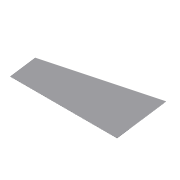
# Autodesk Inventor part: panelBflat_SA
Saved by Autodesk Inventor 2016 (Build 200138000, 138)
## iProperties
Created: 2015-02-12
Part Number: panelBflat_SA
Material: Generic
Document SubType Name: Modeling
Designer: Dave
Density: 1 g/cm^3
Appearance: Default
Author: Dave
Autodesk Inventor part; units mm, degrees
ref_plane "YZ Plane" through (0, 0, 0) normal (1, 0, 0) x (0, 1, 0)
ref_plane "XZ Plane" through (0, 0, 0) normal (0, 1, 0) x (-1, 0, 0)
ref_plane "XY Plane" through (0, 0, 0) normal (0, 0, 1) x (1, 0, 0)
sketch "Sketch1" plane through (0, 0, 0) normal (0, 1, 0) x (-1, 0, 0)
  line L0 (0, 0) -> (-4300, 0) construction
  line L1 (0, 0) -> (-4153.4811, -1112.9219) construction
  line L2 (0, 0) -> (4300, 0) construction
  line L3 (-4300, 0) -> (-4200, 0) construction
  line L4 (-2006.9086, 50) -> (-4293.6038, 50)
  line L5 (-4153.4811, -1112.9219) -> (-3780.7254, -1112.9219) construction
  line L6 (-1925.5839, -567.7225) -> (-4134.3619, -1159.5627)
  line L7 (-1925.5839, -567.7225) -> (-2006.9086, 50)
  line L8 (-4293.6038, 50) -> (-4134.3619, -1159.5627)
  dimension "d0" = 4300
  dimension "d1" = 4300
  dimension "d2" = 165
  dimension "d5" = 50
  dimension "d7" = 50
  dimension "d11" = 1220
  constraints: 20 end point, 4 horizontal, 3 parallel, 1 equal length
  measures "d0" distance of L0.start L0.end
  measures "d1" distance of L0.start L1.end
  measures "d2" angle of L1 L2
  measures "d5" distance between parallel lines of L4 L0
  measures "d7" distance between parallel lines of L6 L1
  measures "d11" distance of L4.end L6.end
extrude "Extrusion1" add sketch "Sketch1" along normal blind 1
body "Solid1"
